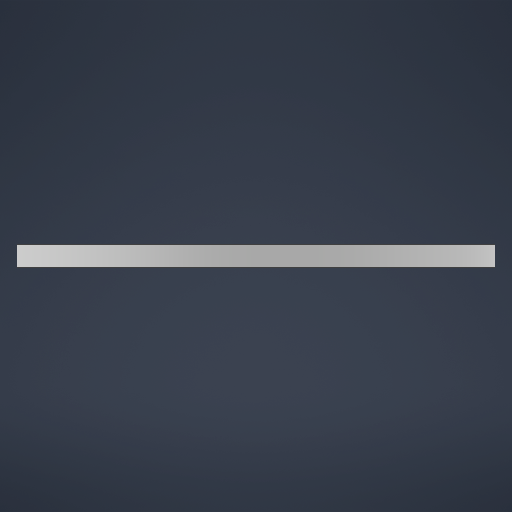
# Autodesk Inventor part: 260mm Housing 1
Saved by Autodesk Inventor 2025 (Build 290162000, 162)
## iProperties
Created: 2024-10-30
Part Number: 260mm Housing 1
Material: Generic
Document SubType Name: Modeling
Designer: mayhe
Density: 1 g/cm^3
Appearance: Default
Author: mayhe
Autodesk Inventor part; units mm, degrees
ref_plane "YZ Plane" through (0, 0, 0) normal (1, 0, 0) x (0, 1, 0)
ref_plane "XZ Plane" through (0, 0, 0) normal (0, 1, 0) x (-1, 0, 0)
ref_plane "XY Plane" through (0, 0, 0) normal (0, 0, 1) x (1, 0, 0)
sketch "Sketch1" plane through (0, 0, 0) normal (0, 1, 0) x (-1, 0, 0)
  circle A0 centre (0, 0) radius 150
  circle A1 centre (0, 0) radius 110
  circle A2 centre (0, 0) radius 130.125
  circle A3 centre (0, 0) radius 140
  circle A4 centre (-140, 0) radius 2.75
  line L0 (-144.0625, 2.3455) -> (-140, 4.691)
  line L1 (-140, 4.691) -> (-135.9375, 2.3455)
  line L2 (-135.9375, 2.3455) -> (-135.9375, -2.3455)
  line L3 (-135.9375, -2.3455) -> (-140, -4.691)
  line L4 (-140, -4.691) -> (-144.0625, -2.3455)
  line L5 (-144.0625, -2.3455) -> (-144.0625, 2.3455)
  circle A5 centre (-113.2624, -82.2899) radius 2.75
  line L6 (-117.9277, -82.7803) -> (-116.0197, -78.4949)
  line L7 (-116.0197, -78.4949) -> (-111.3544, -78.0045)
  line L8 (-111.3544, -78.0045) -> (-108.5971, -81.7996)
  line L9 (-108.5971, -81.7996) -> (-110.5051, -86.085)
  line L10 (-110.5051, -86.085) -> (-115.1704, -86.5754)
  line L11 (-115.1704, -86.5754) -> (-117.9277, -82.7803)
  circle A6 centre (-43.2624, -133.1479) radius 2.75
  line L12 (-46.7484, -136.2868) -> (-47.7238, -131.6983)
  line L13 (-47.7238, -131.6983) -> (-44.2377, -128.5595)
  line L14 (-44.2377, -128.5595) -> (-39.7763, -130.009)
  line L15 (-39.7763, -130.009) -> (-38.801, -134.5975)
  line L16 (-38.801, -134.5975) -> (-42.2871, -137.7364)
  line L17 (-42.2871, -137.7364) -> (-46.7484, -136.2868)
  circle A7 centre (43.2624, -133.1479) radius 2.75
  line L18 (42.2871, -137.7364) -> (38.801, -134.5975)
  line L19 (38.801, -134.5975) -> (39.7763, -130.009)
  line L20 (39.7763, -130.009) -> (44.2377, -128.5595)
  line L21 (44.2377, -128.5595) -> (47.7238, -131.6983)
  line L22 (47.7238, -131.6983) -> (46.7484, -136.2868)
  line L23 (46.7484, -136.2868) -> (42.2871, -137.7364)
  circle A8 centre (113.2624, -82.2899) radius 2.75
  line L24 (115.1704, -86.5754) -> (110.5051, -86.085)
  line L25 (110.5051, -86.085) -> (108.5971, -81.7996)
  line L26 (108.5971, -81.7996) -> (111.3544, -78.0045)
  line L27 (111.3544, -78.0045) -> (116.0197, -78.4949)
  line L28 (116.0197, -78.4949) -> (117.9277, -82.7803)
  line L29 (117.9277, -82.7803) -> (115.1704, -86.5754)
  circle A9 centre (140, 0) radius 2.75
  line L30 (144.0625, -2.3455) -> (140, -4.691)
  line L31 (140, -4.691) -> (135.9375, -2.3455)
  line L32 (135.9375, -2.3455) -> (135.9375, 2.3455)
  line L33 (135.9375, 2.3455) -> (140, 4.691)
  line L34 (140, 4.691) -> (144.0625, 2.3455)
  line L35 (144.0625, 2.3455) -> (144.0625, -2.3455)
  circle A10 centre (113.2624, 82.2899) radius 2.75
  line L36 (117.9277, 82.7803) -> (116.0197, 78.4949)
  line L37 (116.0197, 78.4949) -> (111.3544, 78.0045)
  line L38 (111.3544, 78.0045) -> (108.5971, 81.7996)
  line L39 (108.5971, 81.7996) -> (110.5051, 86.085)
  line L40 (110.5051, 86.085) -> (115.1704, 86.5754)
  line L41 (115.1704, 86.5754) -> (117.9277, 82.7803)
  circle A11 centre (43.2624, 133.1479) radius 2.75
  line L42 (46.7484, 136.2868) -> (47.7238, 131.6983)
  line L43 (47.7238, 131.6983) -> (44.2377, 128.5595)
  line L44 (44.2377, 128.5595) -> (39.7763, 130.009)
  line L45 (39.7763, 130.009) -> (38.801, 134.5975)
  line L46 (38.801, 134.5975) -> (42.2871, 137.7364)
  line L47 (42.2871, 137.7364) -> (46.7484, 136.2868)
  circle A12 centre (-43.2624, 133.1479) radius 2.75
  line L48 (-42.2871, 137.7364) -> (-38.801, 134.5975)
  line L49 (-38.801, 134.5975) -> (-39.7763, 130.009)
  line L50 (-39.7763, 130.009) -> (-44.2377, 128.5595)
  line L51 (-44.2377, 128.5595) -> (-47.7238, 131.6983)
  line L52 (-47.7238, 131.6983) -> (-46.7484, 136.2868)
  line L53 (-46.7484, 136.2868) -> (-42.2871, 137.7364)
  circle A13 centre (-113.2624, 82.2899) radius 2.75
  line L54 (-115.1704, 86.5754) -> (-110.5051, 86.085)
  line L55 (-110.5051, 86.085) -> (-108.5971, 81.7996)
  line L56 (-108.5971, 81.7996) -> (-111.3544, 78.0045)
  line L57 (-111.3544, 78.0045) -> (-116.0197, 78.4949)
  line L58 (-116.0197, 78.4949) -> (-117.9277, 82.7803)
  line L59 (-117.9277, 82.7803) -> (-115.1704, 86.5754)
  point P0 (-144.0625, 0)
  point P1 (-116.549, -84.6778)
  point P2 (-44.5178, -137.0116)
  point P3 (44.5178, -137.0116)
  point P4 (116.549, -84.6778)
  point P5 (144.0625, 0)
  point P6 (116.549, 84.6778)
  point P7 (44.5178, 137.0116)
  point P8 (-44.5178, 137.0116)
  point P9 (-116.549, 84.6778)
  dimension "d20" = 280
  dimension "d0" = 300
  dimension "d1" = 220
  dimension "d19" = 260.25
  dimension "d21" = 5.5
  dimension "d25" = 360
  constraints: 120 end point, 13 centre point, 7 coincident, 1 horizontal alignment, 1 midpoint, 176 other
  measures "d0" diameter of A0
  measures "d1" diameter of A1
  measures "d19" diameter of A2
  measures "d21" diameter of A4
extrude "Extrusion1" add sketch "Sketch1" along normal blind 2 contours A0 | A2 | A9 A3 L31 L32 L33 | A3 L33 L34 L35 L30 L31 A9 | L33 L32 L31 A3 L27 L26 L25 L21 L20 L19 L15 L14 L13 L9 L8 L7 L3 L2 L1 L57 L56 L55 L51 L50 L49 L45 L44 L43 L39 L38 L37 | L37 L38 L39 A3 A10 | A3 A10 L39 L40 L41 L36 L37 | L27 L28 L29 L24 L25 A3 A8 | A3 A8 L25 L26 L27 | L43 L44 L45 A3 A11 | A3 A11 L45 L46 L47 L42 L43 | L21 L22 L23 L18 L19 A3 A7 | A3 A7 L19 L20 L21 | L49 L50 L51 A3 A12 | A3 A12 L51 L52 L53 L48 L49 | L15 L16 L17 L12 L13 A3 A6 | A3 A6 L13 L14 L15 | L55 L56 L57 A3 A13 | A3 A13 L57 L58 L59 L54 L55 | L9 L10 L11 L6 L7 A3 A5 | A3 A5 L7 L8 L9 | L1 L2 L3 A3 A4 | A3 A4 L3 L4 L5 L0 L1
extrude "Extrusion3" add sketch "Sketch1" along normal blind 4.25 contours A0 | A2 | L33 L32 L31 A3 L27 L26 L25 L21 L20 L19 L15 L14 L13 L9 L8 L7 L3 L2 L1 L57 L56 L55 L51 L50 L49 L45 L44 L43 L39 L38 L37
sketch "Sketch4" plane through (0, 4.25, 0) normal (0, 1, 0) x (1, 0, 0)
  circle A0 centre (0, 0) radius 110
  circle A1 centre (0, 0) radius 150
  circle A2 centre (-140, 0) radius 2.75 projected
  circle A3 centre (-140, 0) radius 2.75
  circle A4 centre (0, 0) radius 140
  circle A5 centre (-113.2624, -82.2899) radius 2.75
  circle A6 centre (-43.2624, -133.1479) radius 2.75
  circle A7 centre (43.2624, -133.1479) radius 2.75
  circle A8 centre (113.2624, -82.2899) radius 2.75
  circle A9 centre (140, 0) radius 2.75
  circle A10 centre (113.2624, 82.2899) radius 2.75
  circle A11 centre (43.2624, 133.1479) radius 2.75
  circle A12 centre (-43.2624, 133.1479) radius 2.75
  circle A13 centre (-113.2624, 82.2899) radius 2.75
  dimension "d31" = 360
  constraints: 12 centre point, 4 coincident, 1 horizontal alignment, 23 other
extrude "Extrusion4" add sketch "Sketch4" along normal blind 10.75 contours A1 | A2 A4 A13 A12 A11 A10 A9 A8 A7 A6 A5
sketch "Sketch3" plane through (0, 15, 0) normal (0, 1, 0) x (1, 0, 0)
  circle A0 centre (0, 0) radius 125
  circle A1 centre (0, 125) radius 2.75
  circle A2 centre (-73.4732, 101.1271) radius 2.75
  circle A3 centre (-118.8821, 38.6271) radius 2.75
  circle A4 centre (-118.8821, -38.6271) radius 2.75
  circle A5 centre (-73.4732, -101.1271) radius 2.75
  circle A6 centre (0, -125) radius 2.75
  circle A7 centre (73.4732, -101.1271) radius 2.75
  circle A8 centre (118.8821, -38.6271) radius 2.75
  circle A9 centre (118.8821, 38.6271) radius 2.75
  circle A10 centre (73.4732, 101.1271) radius 2.75
  circle A11 centre (0, 0) radius 130.125
  dimension "d13" = 250
  dimension "d14" = 5.5
  dimension "d17" = 360
  dimension "d35" = 260.25
  constraints: 11 centre point, 2 coincident, 1 vertical alignment, 23 other
  measures "d14" diameter of A1
  measures "d35" diameter of A11
extrude "Extrusion5" cut sketch "Sketch3" against normal blind 2.125 contours A0 A8 A7 A6 A5 A4 A3 A2 A1 A10 A9 | A11
hole "Hole1" at (-118.8821, 15, 38.6271) at (-73.4732, 15, 101.1271) at (0, 15, 125) at (73.4732, 15, 101.1271) at (118.8821, 15, 38.6271) at (118.8821, 15, -38.6271) at (73.4732, 15, -101.1271) at (0, 15, -125) at (-73.4732, 15, -101.1271) at (-118.8821, 15, -38.6271) direction (0, -1, 0) diameter 5.5 end through all counterbore diameter 10.475 counterbore depth 7.375
sketch "Sketch5" plane through (0, 0, 0) normal (1, 0, 0) x (0, 1, 0)
  line L0 (12.875, 130.1203) -> (12.875, 105.9171) projected
  line L1 (0, -150) -> (0, 150) projected
  line L2 (13.875, 113.5) -> (11.875, 113.5)
  line L3 (11.875, 113.5) -> (11.875, 115.5)
  line L4 (11.875, 115.5) -> (13.875, 115.5)
  line L5 (13.875, 115.5) -> (13.875, 113.5)
  line L6 (13.875, 113.5) -> (11.875, 115.5) construction
  line L7 (11.875, 113.5) -> (13.875, 115.5) construction
  line L8 (12.875, 110) -> (0, 110) projected
  line L9 (12.875, 110) -> (0, 110)
  line L10 (1, 115.5) -> (-1, 115.5)
  line L11 (-1, 115.5) -> (-1, 113.5)
  line L12 (-1, 113.5) -> (1, 113.5)
  line L13 (1, 113.5) -> (1, 115.5)
  line L14 (1, 115.5) -> (-1, 113.5) construction
  line L15 (-1, 115.5) -> (1, 113.5) construction
  line L16 (-4.2, 0) -> (18.2, 0) projected
  point P0 (0, 0)
  point P1 (12.875, 114.5)
  point P2 (0, 114.5)
  dimension "d45" = 2
  dimension "d46" = 2
  dimension "d48" = 4.5
  dimension "d49" = 2
  dimension "d50" = 2
  constraints: 26 end point, 5 point on line, 4 midpoint, 4 parallel, 2 horizontal, 2 perpendicular, 2 vertical alignment
  measures "d45" distance of L3.end L4.end
  measures "d46" distance of L2.end L3.end
  measures "d48" distance from line of L8 point (12.875, 114.5)
  measures "d49" distance of L12.end L11.end
  measures "d50" distance of L11.end L10.end
revolve "Revolution1" cut sketch "Sketch5" angle 360 about axis through (0, -10, 0) along (0, 1, 0)
body "Solid1"
